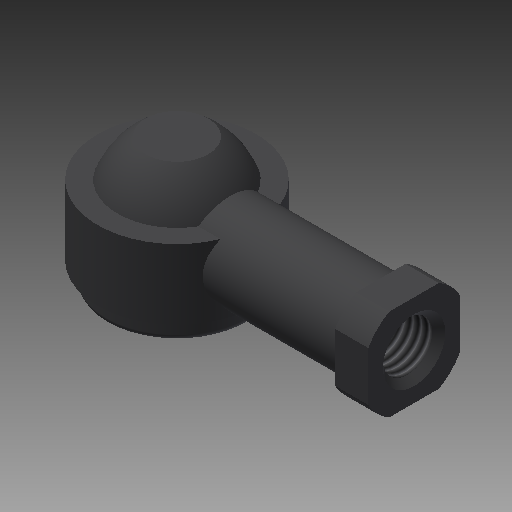
# Autodesk Inventor part: LHSA 14 Body1
Saved by Autodesk Inventor 2018 (Build 220112000, 112)
## iProperties
Category: PARTsolutions
Company: IKO
Created: 2017-09-07
Part Number: LHSA 14 Body1
Catalog Web Link: www.cadenas.de
Description: LHSA B1-
Vendor: IKO
Document SubType Name: Modeling
Designer: psAdmin
Manufacturer: IKO
Mass: 24.1498 g
Surface Area: 124.326 cm^2
Volume: 24.1498 cm^3
Density: 1 g/cm^3
Material: 一般
Appearance: PSOLRGB-128-128-128
PSOL_IDENT_0: {$CADENAS_DATA\23d-libs\iko\iko_bearings\l_balls\lhsa_body.prj},169 {VTYP=3D},{NB=LHSA 14 Body1},{LI
PSOL_IDENT_1: NA=LHSA 14 Body1},{NN=LHSA B1},{DATE=13.10.2016 10:02:12},{GEOMDATE=06.12.2007 08:55:00},{VERSION=},
PSOL_IDENT_2: {LINEID=90},{LINESUBID=-1},{WBVAR=}  {NB=LHSA 14 Body1},{LINA=LHSA 14 Body1},{KT=DUMMY},{IDNR=},{ORD
PSOL_IDENT_3: ER=LHSA 14},{VERS=3},{RID=G_80},{STDRT=14},{DESCR=LHSA},{TRNUMBER=},{PAST=A},{REST=O},{MASS=260},{S=
PSOL_IDENT_4: M14x2},{KDM=11.835},{NDM=14.000},{P1=2.000},{V=14},{D=38},{L=76.0},{L1=57},{L2=30},{SL1=8.0},{W=22},
PSOL_IDENT_5: {W1=22},{W2=22},{D1=20.0},{D2=25},{LL=72.0},{P=17.0},{LL1=22.5},{LL2=33.5},{LL3=22.0},{SDK=25.400},{
PSOL_IDENT_6: V1=15.0},{D3=15.0000},{D4=28.2138},{D5=34.0},{D6=34.00},{L3=71.2350},{L4=35.1132},{L5=38.0},{L12=39.
PSOL_IDENT_7: 3932},{B=12.0},{B1=7.0},{B2=12.0},{B3=15.0},{B4=16.8},{B5=21.8000},{LL4=8.5},{LL5=12.7},{CB=0.0},{CC=
PSOL_IDENT_8: 1.0},{E=0},{F=0.0},{C1=1.5825},{C2=2.0},{R1=5},{R2=50.6010},{R3=20.0},{R4=1.5},{CS=14600},{SS1=11.54
PSOL_IDENT_9: 6},{S1=14},{LX=32},{LX1=36.6},{BL=3},{SC=1}
NN: LHSA B1
NB: LHSA 14 Body1
NBSYN: $ORDER. Body1
LINA: LHSA 14 Body1
ORDER: LHSA 14
VERS: 3
RID: G_80
STDRT: 14
DESCR: LHSA
PAST: A
REST: O
MASS: 260
S: M14x2
NDM: 14.000
P1: 2.000
V: 14
D: 38
L: 76.0
L1: 57
L2: 30
SL1: 8.0
W: 22
W1: 22
W2: 22
D1: 20.0
D2: 25
LL: 72.0
P: 17.0
LL1: 22.5
LL2: 33.5
LL3: 22.0
SDK: 25.400
V1: 15.0
D3: 15.0000
D4: 28.2138
D5: 34.0
D6: 34.00
L3: 71.2350
L4: 35.1132
L5: 38.0
L12: 39.3932
B: 12.0
B1: 7.0
B2: 12.0
B3: 15.0
B4: 16.8
B5: 21.8000
LL4: 8.5
LL5: 12.7
CB: 0.0
CC: 1.0
E: 0
F: 0.0
C1: 1.5825
C2: 2.0
R1: 5
R2: 50.6010
R3: 20.0
R4: 1.5
CS: 14600
SS1: 11.546
S1: 14
LX: 32
LX1: 36.6
BL: 3
SC: 1
SUPPLIER: IKO
ARTICLENO: LHSA 14 Body1
BOMINFO: LHSA 14 Body1
CREATOR: CADENAS GmbH
Title: LHSA 14 Body1
Author: Cadenas PARTsolutions
Autodesk Inventor part; units mm, degrees
sketch "Sketch_2" plane through (0, 0, 0) normal (0, 0, 1) x (1, 0, 0)
  line L0 (57, 22.5) -> (0, 22.5)
  line L1 (0, 22.5) -> (0, 32.5)
  line L2 (0, 32.5) -> (49, 32.5)
  line L3 (49, 32.5) -> (49, 35)
  line L4 (49, 35) -> (57, 35)
  line L5 (57, 35) -> (57, 22.5)
  line L6 (57, 22.5) -> (0, 22.5)
  constraints: 14 end point
revolve "Revolution1" add sketch "Sketch_2" angle 360 about axis through (57, 22.5, 0) along (1, 0, 0)
sketch "Sketch_16" plane through (0, 0, 0) normal (0, 0, 1) x (1, 0, 0)
  line L0 (-19, 17.5) -> (-19, 7.5)
  line L1 (-19, 7.5) -> (60.8, 7.5)
  line L2 (60.8, 7.5) -> (60.8, 37.5)
  line L3 (60.8, 37.5) -> (21.8868, 37.5)
  line L4 (21.8868, 37.5) -> (21.8868, 32.5)
  line L5 (21.8868, 32.5) -> (49, 32.5)
  line L6 (49, 32.5) -> (49, 33.5)
  line L7 (49, 33.5) -> (57, 33.5)
  line L8 (57, 33.5) -> (57, 11.5)
  line L9 (57, 11.5) -> (49, 11.5)
  line L10 (49, 11.5) -> (49, 12.5)
  line L11 (49, 12.5) -> (21.8868, 12.5)
  line L12 (21.8868, 12.5) -> (19, 17.5)
  line L13 (19, 17.5) -> (-19, 17.5)
  constraints: 28 end point
extrude "Extrusion1" cut sketch "Sketch_16" along normal mid plane 50
sketch "Sketch_12" plane through (0, 0, 0) normal (0, 0, 1) x (1, 0, 0)
  line L0 (0, 14.5) -> (0, 38.5)
  line L1 (0, 38.5) -> (7.5, 38.5)
  arc A0 (14.235, 29.5) -> (7.5, 38.5) centre (-4.5, 22.5) ccw
  line L2 (14.235, 29.5) -> (19, 29.5)
  line L3 (19, 29.5) -> (19, 17.5)
  line L4 (19, 17.5) -> (17, 17.5)
  line L5 (17, 17.5) -> (17, 14.5)
  line L6 (17, 14.5) -> (0, 14.5)
  line L7 (0, 14.5) -> (0, 38.5)
  constraints: 16 end point, 2 point on circle, 1 centre point
revolve "Revolution2" add sketch "Sketch_12" angle 360 about axis through (0, 14.5, 0) along (0, -1, 0)
sketch "Sketch_13" plane through (0, 0, 0) normal (0, 0, 1) x (1, 0, 0)
  line L0 (12.7, 22.5) -> (-12.7, 22.5)
  arc A0 (12.7, 22.5) -> (-12.7, 22.5) centre (0, 22.5) ccw
  line L1 (12.7, 22.5) -> (-12.7, 22.5)
  constraints: 4 end point, 2 point on circle, 1 centre point
revolve "Revolution3" cut sketch "Sketch_13" angle 360 about axis through (12.7, 22.5, 0) along (1, 0, 0)
sketch "Sketch_14" plane through (0, 0, 0) normal (0, 0, 1) x (1, 0, 0)
  line L0 (0, 14.5) -> (0, 17.5)
  line L1 (0, 17.5) -> (14.1069, 17.5)
  line L2 (14.1069, 17.5) -> (14.1069, 14.5)
  line L3 (14.1069, 14.5) -> (0, 14.5)
  line L4 (0, 14.5) -> (0, 17.5)
  constraints: 10 end point
revolve "Revolution4" cut sketch "Sketch_14" angle 360 about axis through (0, 14.5, 0) along (0, -1, 0)
sketch "Sketch_15" plane through (0, 0, 0) normal (0, 0, 1) x (1, 0, 0)
  line L0 (0, 14.5) -> (0, 17.5)
  line L1 (9.8636, 14.5) -> (14.1069, 14.5)
  line L2 (14.1069, 14.5) -> (14.1069, 17.5)
  line L3 (14.1069, 17.5) -> (11.6743, 17.5)
  arc A0 (9.8636, 14.5) -> (11.6743, 17.5) centre (0, 22.5) ccw
  constraints: 8 end point, 2 point on circle, 1 centre point
revolve "Revolution5" add sketch "Sketch_15" angle 360 about axis through (0, 14.5, 0) along (0, -1, 0)
sketch "Sketch_17" plane through (0, 0, 0) normal (0, 0, 1) x (1, 0, 0)
  line L0 (0, 8.5) -> (0, 17.5)
  line L1 (7.5, 9.5) -> (7.5, 8.5)
  line L2 (7.5, 8.5) -> (8.5, 8.5)
  line L3 (8.5, 8.5) -> (15.5, 7.7)
  arc A0 (15.5, 7.7) -> (17, 9.2) centre (15.5, 9.2) ccw
  line L4 (17, 9.2) -> (17, 12.7)
  line L5 (17, 12.7) -> (19, 12.7)
  line L6 (19, 12.7) -> (19, 17.5)
  line L7 (19, 17.5) -> (17, 17.5)
  line L8 (17, 17.5) -> (17, 14.5)
  line L9 (17, 14.5) -> (16, 14.5)
  line L10 (16, 14.5) -> (16, 10.2)
  arc A1 (14.5, 8.7) -> (16, 10.2) centre (14.5, 10.2) ccw
  line L11 (14.5, 8.7) -> (8.5, 9.5)
  line L12 (8.5, 9.5) -> (7.5, 9.5)
  constraints: 26 end point, 4 point on circle, 2 centre point
revolve "Revolution6" add sketch "Sketch_17" angle 360 about axis through (0, 8.5, 0) along (0, -1, 0)
sketch "Sketch8" plane through (57, 22.5, 0) normal (1, 0, 0) x (0, 0, -1)
  point P0 (0, 0)
hole "Hole1" at (57, 22.5, 0) direction (-1, 0, 0) diameter 11.835 depth 33.5825 tip angle 120 countersink diameter 15 countersink angle 90 thread size "M14x2" class "6H" standard "ISO Metric profile"
sketch "Sketch_20" plane through (49, 0, 0) normal (1, 0, 0) x (0, 0, -1)
  line L0 (-16.5, 9.3) -> (16.5, 9.3)
  line L1 (16.5, 9.3) -> (16.5, 35.7)
  line L2 (16.5, 35.7) -> (-16.5, 35.7)
  line L3 (-16.5, 35.7) -> (-16.5, 9.3)
  line L4 (-11, 33.5) -> (-11, 11.5)
  line L5 (-11, 11.5) -> (11, 11.5)
  line L6 (11, 11.5) -> (11, 33.5)
  line L7 (11, 33.5) -> (-11, 33.5)
  constraints: 16 end point
extrude "Extrusion2" cut sketch "Sketch_20" along normal blind 8
ref_plane "IP1_XY" through (0, 22.5, 0) normal (0, 0, 1) x (1, 0, 0)
ref_plane "IP1_YZ" through (0, 22.5, 0) normal (1, 0, 0) x (0, 1, 0)
ref_plane "IP1_ZX" through (0, 22.5, 0) normal (0, 1, 0) x (0, 0, 1)
body "Solid1"
